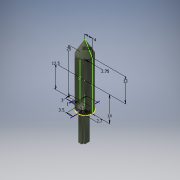
# Autodesk Inventor part: Rotator Frame_xw
Saved by Autodesk Inventor 2016 (Build 200138000, 138)
## iProperties
Created: 2014-06-20
Part Number: Rotator Frame_xw
Document SubType Name: Modeling
Designer: 121767
Density: 1.068 g/cm^3
Material: SAN Plastic
Appearance: Precast Smooth
Author: 121767
Autodesk Inventor part; units mm, degrees
ref_plane "YZ Plane" through (0, 0, 0) normal (1, 0, 0) x (0, 1, 0)
ref_plane "XZ Plane" through (0, 0, 0) normal (0, 1, 0) x (-1, 0, 0)
ref_plane "XY Plane" through (0, 0, 0) normal (0, 0, 1) x (1, 0, 0)
sketch "Sketch1" plane through (0, 0, 0) normal (0, 0, 1) x (1, 0, 0)
  line L0 (0, 19.9282) -> (4, 13)
  line L1 (4, 13) -> (4, -14)
  line L2 (4, -14) -> (0, -14)
  line L3 (0, -25.9015) -> (0, 19.9282)
  line L4 (2.75, -12.5) -> (-2.75, -12.5)
  line L5 (-2.75, -12.5) -> (-2.75, 12.5)
  line L6 (-2.75, 12.5) -> (2.75, 12.5)
  line L7 (2.75, 12.5) -> (2.75, -12.5)
  point P0 (0, 0)
  dimension "d0" = 30
  dimension "d1" = 4
  dimension "d41" = 25
  dimension "d45" = 14
  dimension "d46" = 12.5
  dimension "d47" = 2.75
  dimension "d48" = 13
  constraints: 16 end point, 2 parallel, 2 perpendicular, 1 horizontal, 1 point on line, 1 vertical, 1 other
  measures "d0" angle of L3 L0
  measures "d1" distance between parallel lines of L1 L3
  measures "d41" distance between parallel lines of L6 L4
  measures "d45" distance from line of L2 point (0, 0)
  measures "d46" distance from line of point (0, 0) L4
  measures "d47" distance between parallel lines of L7 L3
  measures "d48" vertical distance of point (0, 0) L0.end
revolve "main cylinder" add sketch "Sketch1" angle 360 about axis through (0, -25.9015, 0) along (0, 1, 0) contours L0 L1 L2 L3 L4 L7 L6 | L6 L7 L4 L3
extrude "main window" cut sketch "Sketch1" against normal mid plane 25.4 contours L6 L7 L4 L3 | L3 L4 L5 L6
sketch "Sketch2" plane through (-2.75, -12.5, 2.9047) normal (1, 0, 0) x (0, 0, -1)
  point P0 (2.9047, 12.5)
  point P1 (2.9047, 12.5)
  constraints: 1 coincident
hole "full side hole" at (-2.75, 0, 0) direction (-1, 0, 0) diameter 1 depth 25.4
sketch "Sketch3" plane through (0, -14, 0) normal (0, -1, 0) x (1, 0, 0)
  circle A0 centre (0, 0) radius 2.5 projected
  circle A1 centre (0, 0) radius 4 projected
  line L0 (-3.9686, 0.5) -> (-3.5, 0.5)
  line L1 (-3.5, 0.5) -> (-3.5, -0.5)
  line L2 (-3.5, -0.5) -> (-3.9686, -0.5)
  line L3 (-10.1288, 0) -> (5.4225, 0)
  line L4 (0, 8.0973) -> (0, -8.0973)
  line L5 (-2.9513, 2.7) -> (2.9513, 2.7)
  arc A2 (3.5536, -1.8362) -> (-3.5536, -1.8362) centre (0, -7) ccw
  line L6 (3.9686, 0.5) -> (3.5, 0.5)
  line L7 (3.5, 0.5) -> (3.5, -0.5)
  line L8 (3.5, -0.5) -> (3.9686, -0.5)
  line L9 (1.75, -0.956) -> (-1.75, -0.956)
  line L10 (-1.75, -0.956) -> (-1.75, 1.7854)
  line L11 (-1.75, 2.7) -> (-0.988, 2.7) construction
  line L12 (1.75, 2.7) -> (1.75, 2.4638) construction
  line L13 (0.988, 2.7) -> (0.988, 1.7526)
  line L14 (0.988, 1.7526) -> (1.75, 1.7526)
  line L15 (-0.988, 2.7) -> (-0.988, 1.7526)
  line L16 (-0.988, 1.7526) -> (-1.75, 1.7526)
  line L17 (1.75, 1.7854) -> (1.75, -0.956)
  line L18 (1.75, 2.4638) -> (1.75, 1.7854) construction
  line L19 (-1.75, 1.7854) -> (-1.75, 2.4638) construction
  line L20 (-1.75, 2.4638) -> (-1.75, 2.7) construction
  line L21 (0.988, 2.7) -> (1.75, 2.7) construction
  line L22 (-0.988, 2.7) -> (0.988, 2.7)
  point P0 (0, -3)
  dimension "d14" = 1
  dimension "d15" = 3.5
  dimension "d20" = 3
  dimension "d35" = 2.7
  dimension "d38" = 7
  dimension "d75" = 3.5
  dimension "d78" = 1.7526
  dimension "d79" = 0.762
  constraints: 46 end point, 16 parallel, 10 perpendicular, 10 point on line, 5 collinear, 4 point on circle, 2 horizontal, 2 midpoint, 1 centre point, 1 coincident, 1 vertical, 12 other
  measures "d14" distance between parallel lines of L2 L0
  measures "d15" distance from line of A0.centre L1
  measures "d20" distance from line of L3 point (0, -3)
  measures "d35" distance between parallel lines of L3 L5
  measures "d38" distance from line of point (0, -7) L3
  measures "d75" distance between parallel lines of L10 L12
  measures "d78" distance between parallel lines of L3 L14
  measures "d79" distance of L13.end L14.end
hole "partial side hole" at (-2.75, 0, 0) direction (-1, 0, 0) diameter 2 depth 0.75
extrude "side channels" cut sketch "Sketch3" against normal blind 14.5 contours L7 L6 A1 L3 | L3 A1 L8 L7 | L3 A1 L0 L1 | L1 L2 A1 L3
hole "thread hole" at (0, -14, -3) direction (0, 1, 0) diameter 1 end through all
extrude "Extrusion4" cut sketch "Sketch3" against normal blind 10 contours L5 L4 A1 | L5 A1 L4
extrude "Extrusion5" cut sketch "Sketch3" along normal blind 20 contours A2 A1 L4 A0 | A0 L4 L9 A2 | L4 A1 A2 A0 | A0 A2 L9 L4 | L9 L4 A2 | L9 A2 L4
extrude "Extrusion6" add sketch "Sketch3" along normal blind 15 contours L17 L9 A2 L4 L3 | L3 L4 A0 L13 L14 L17 | A0 L4 L5 L13 | L9 L4 A2 | L4 A2 L9 L10 L3 | L3 L10 L16 L15 A0 L4 | A0 L15 L5 L4 | L9 A2 L4
fillet "Fillet1" radius 2 4 edges at (-2.75, 12.5, 0) (2.75, 12.5, 0) (-2.75, -12.5, -0.1024) (2.75, -12.5, -0.1024)
mirror "Mirror4" about plane through (0, 0, 0) normal (1, 0, 0) of "partial side hole", "full side hole"
body "Solid1"
